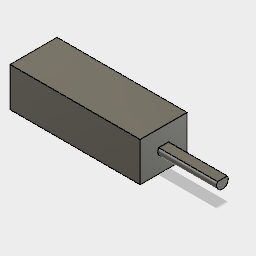
_FYP_Project.e5b741b6-de03-4121-ac4c-455f43841e72 (Autodesk Fusion 360 design; units mm, degrees)
Autodesk Fusion 360 part; units mm, degrees
note: some values were not read from the file. Chosen so that the rebuilt part matches the saved one: which face or edge a step refers to. Set by a fixed rule: which sketch regions a step uses.
sketch "Sketch1" plane through (0, 0, 0) normal (1, 0, 0) x (0, 0, -1)
  circle A0 centre (0, 0) radius 40
  line L0 (-2.9, 1.75) -> (2.9, 1.75)
  line L1 (2.9, 1.75) -> (2.9, -1.75)
  line L2 (2.9, -1.75) -> (-2.9, -1.75)
  line L3 (-2.9, -1.75) -> (-2.9, 1.75)
  line L4 (-2.9, 1.75) -> (2.9, -1.75) construction
  line L5 (2.9, 1.75) -> (-2.9, -1.75) construction
  dimension "d1" = 80
  dimension "d2" = 5.8
  dimension "d3" = 3.5
  measures "d1" diameter of A0
  measures "d2" distance of L1.end L2.end
  measures "d3" distance of L0.end L1.end
sketch "Sketch2" plane through (0, 0, 0) normal (0, 1, 0) x (1, 0, 0)
  line L0 (16.6, 6) -> (-16.6, 6)
  line L1 (-16.6, 6) -> (-16.6, -6)
  line L2 (-16.6, -6) -> (16.6, -6)
  line L3 (16.6, -6) -> (16.6, 6)
  line L4 (16.6, 6) -> (-16.6, -6) construction
  line L5 (-16.6, 6) -> (16.6, -6) construction
  dimension "d6" = 33.2
  dimension "d7" = 12
  measures "d6" distance of L1.end L2.end
  measures "d7" distance of L0.end L1.end
extrude "Extrude2" add sketch "Sketch2" along normal blind 10 makes body 1
sketch "Sketch3" plane through (16.6, 0, 0) normal (1, 0, 0) x (0, 0, -1)
  line L0 (-6, 0) -> (6, 0)
  line L1 (6, 0) -> (6, 10)
  line L2 (6, 10) -> (-6, 10)
  line L3 (-6, 10) -> (-6, 0)
  circle A0 centre (-0.0016, 5.0186) radius 1.5
  line L4 (-1.2598, 5.8353) -> (1.2566, 5.8353)
  dimension "d10" = 3
  measures "d10" diameter of A0
extrude "Extrude3" add sketch "Sketch3" along normal blind 15 contours A0 L4 picked at (0.569, 4.736) bodies 1
sketch "Sketch4" plane through (0, 0, 0) normal (1, 0, 0) x (0, 0, -1)
  circle A0 centre (0, 0) radius 30
  dimension "d13" = 60
  measures "d13" diameter of A0
extrude "Extrude4" add sketch "Sketch4" along normal blind 8 separate body makes body 2
sketch "Sketch5" plane through (0, 0, 0) normal (-1, 0, 0) x (0, 0, 1)
  circle A0 centre (0, 0) radius 30
  circle A1 centre (0, 0) radius 1.5
  line L0 (-1.26, 0.8139) -> (1.26, 0.8139)
  dimension "d20" = 3
  dimension "d21" = 2.52
  measures "d20" diameter of A1
  measures "d21" distance of L0.start L0.end
extrude "Extrude5" cut sketch "Sketch5" against normal blind 14 contours A1 L0 picked at (-0.4465, 0.3176) bodies 2
copy_body "Body->Comp1" bodies 2 removing the originals makes body 3 in component "Component"
component "Component" placed x (1, 0, 0) y (0, 1, 0) z (0, 0, 1) at (0, 0, 0)
hidden bodies 3
